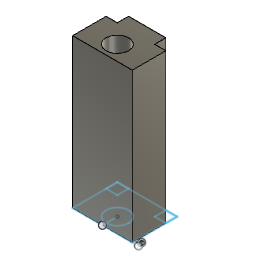
Week 2 HW Drawing 2 (Autodesk Fusion 360 archive; units mm, degrees)
design "Week 2 HW"
Autodesk Fusion 360 part; units mm, degrees
sketch "Object 1 Base" plane through (0, 0, 0) normal (0, 0, 1) x (1, 0, 0)
  line L0 (40, 0) -> (-40, 0)
  line L1 (-40, 0) -> (-40, 60)
  line L2 (-40, 60) -> (40, 60)
  line L3 (40, 60) -> (40, 0)
  line L4 (0, 0) -> (0, 20)
  circle A0 centre (0, 20) radius 15
  line L5 (-40, 60) -> (-25, 60)
  line L6 (-25, 60) -> (-25, 45)
  line L7 (-25, 45) -> (-40, 45)
  line L8 (-40, 45) -> (-40, 60)
  line L9 (40, 60) -> (25, 60)
  line L10 (25, 60) -> (25, 45)
  line L11 (25, 45) -> (40, 45)
  line L12 (40, 45) -> (40, 60)
  dimension "d5" = 80
  dimension "d6" = 60
  dimension "d7" = 20
  dimension "d8" = 30
  dimension "d9" = 15
  dimension "d10" = 15
  dimension "d11" = 15
  dimension "d12" = 15
  constraint horizontal L0
  constraint parallel L0 L2
  constraint parallel L1 L3
  constraint perpendicular L0 L4
  constraint coincident L4.end A0.centre
  constraint horizontal L5
  constraint vertical L6
  constraint horizontal L7
  constraint vertical L8
  constraint horizontal L9
  constraint vertical L10
  constraint horizontal L11
  constraint vertical L12
  measures "d5" distance of L1.end L2.end
  measures "d6" distance of L0.end L1.end
  measures "d7" distance of L4.start L4.end
  measures "d8" diameter of A0
  measures "d9" distance of L1.end L5.end
  measures "d10" distance of L1.end L7.end
  measures "d11" distance of L2.end L9.end
  measures "d12" distance of L2.end L11.end
extrude "Extrude2" add sketch "Object 1 Base" along normal blind 100 contours L0 L1 L2 L3 L6 L7 L10 L11 makes body 1
sketch "Object 2 Base" plane through (0, 0, 0) normal (0, 0, 1) x (1, 0, 0)
  line L0 (45, 0) -> (48.5, 0)
  line L1 (48.5, 0) -> (48.5, 1.375)
  line L2 (48.5, 1.375) -> (45, 1.375)
  line L3 (45, 1.375) -> (45, 0)
  line L4 (45, 1.375) -> (48.5, 1.375)
  line L5 (48.5, 1.375) -> (48.5, 5.875)
  line L6 (48.5, 5.875) -> (45, 5.875)
  line L7 (45, 5.875) -> (45, 1.375)
  circle A0 centre (46.75, 5.875) radius 0.5
  circle A1 centre (46.75, 5.875) radius 1.75
  line L8 (46, 0) -> (47.5, 0)
  line L9 (46.75, 0) -> (46.75, 0.75)
  line L10 (47.5, 0) -> (47.933, 0.75)
  line L11 (47.5, 0) -> (48.366, 0) construction
  line L12 (46, 0) -> (45.567, 0.75)
  line L13 (45.567, 0.75) -> (47.933, 0.75)
  dimension "d17" = 3.5
  dimension "d18" = 1.375
  dimension "d19" = 4.5
  dimension "d20" = 1
  dimension "d21" = 3.5
  dimension "d22" = 1.5
  dimension "d23" = 0.75
  dimension "d24" = 60
  dimension "d25" = 120
  constraint horizontal L0
  constraint vertical L1
  constraint horizontal L2
  constraint vertical L3
  constraint horizontal L4
  constraint vertical L5
  constraint horizontal L6
  constraint vertical L7
  constraint midpoint L6 A0.centre
  constraint concentric A0 A1
  constraint coincident L0 L8.start
  constraint midpoint L0 L8
  constraint midpoint L0 L9.start
  constraint perpendicular L0 L9
  constraint horizontal L11
  constraint perpendicular L9 L13
  measures "d17" distance of L0.start L0.end
  measures "d18" distance of L0.start L2.end
  measures "d19" distance of L2.end L6.end
  measures "d20" diameter of A0
  measures "d21" diameter of A1
  measures "d22" distance of L8.start L8.end
  measures "d23" distance of L9.start L9.end
  measures "d24" angle of L10 L11
  measures "d25" angle of L10 L12
extrude "Extrude4" add sketch "Object 2 Base" along normal blind 2.75 separate body contours L0 L1 L2 L3 L4 L10 L12 L13 makes body 2
extrude "Extrude3" add sketch "Object 2 Base" along normal blind 0.875 separate body contours L0 L1 L2 L3 L4 L10 L12 L13 | L2 L4 L5 L7 A1 | L6 A0 A1 | L6 A0 A1 makes body 3
combine "Combine1" operation add target body 2 tool bodies 3
sketch "Object 2 Surface" plane through (0, 0, 0.875) normal (0, 0, 1) x (-1, 0, 0)
  line L0 (-45, -1.375) -> (-48.5, -1.375)
  line L1 (-48.5, -1.375) -> (-48.5, -5.875)
  arc A0 (-48.5, -5.875) -> (-45, -5.875) centre (-46.75, -5.875) ccw
  line L2 (-45, -5.875) -> (-45, -1.375)
  circle A1 centre (-46.75, -5.875) radius 0.5
  circle A2 centre (-46.75, -5.875) radius 0.875
  dimension "d33" = 1.75
  constraint concentric A0 A2
  measures "d33" diameter of A2
extrude "Extrude6" cut sketch "Object 2 Surface" against normal blind 0.4375 contours A2 bodies 2
extrude "Extrude7" add 1 faces at (-0.2453, 51.6606, 100) along direction (0, 0, 1) blind 100 on bodies 1 bodies 1
extrude "Extrude1" [rolled back] along distance 100 taper angle 0
sketch "Sketch2" plane through (0, 0, 0) normal (0, 1, 0) x (1, 0, 0)
sketch "Sketch3" plane through (0, 0, 0) normal (0, 0, 1) x (1, 0, 0)
named bodies: "Object 1", "Object 2"
